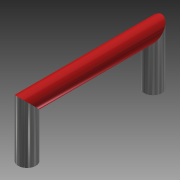
# Autodesk Inventor part: Wire 3
Saved by Autodesk Inventor 2015 (Build 190159000, 159)
## iProperties
Created: 2016-01-20
Part Number: Wire 3
Material: Generic
Document SubType Name: Modeling
Designer: Kyle
Density: 1 g/cm^3
Appearance: Default
Author: Kyle
Autodesk Inventor part; units mm, degrees
ref_plane "YZ Plane" through (0, 0, 0) normal (1, 0, 0) x (0, 1, 0)
ref_plane "XZ Plane" through (0, 0, 0) normal (0, 1, 0) x (-1, 0, 0)
ref_plane "XY Plane" through (0, 0, 0) normal (0, 0, 1) x (1, 0, 0)
sketch "Sketch1" plane through (0, 0, 0) normal (0, 0, 1) x (1, 0, 0)
  line L0 (0, 0) -> (1.0668, 0)
  line L1 (1.0668, 0) -> (1.0668, 1.0668)
  line L2 (1.0668, 1.0668) -> (0, 1.0668)
  line L3 (0, 1.0668) -> (0, 0)
  dimension "d0" = 1.0668
  dimension "d1" = 1.0668
  constraints: 8 end point, 2 parallel, 1 horizontal, 1 perpendicular
  measures "d0" distance of L1.end L2.end
  measures "d1" distance of L0.end L1.end
extrude "Extrusion1" add sketch "Sketch1" along normal blind 8.6868
sketch "Sketch2" plane through (0, 0, 0) normal (0, -1, 0) x (1, 0, 0)
  line L0 (0, 0) -> (0, 8.6868) projected
  line L1 (1.0668, 0) -> (0, 0)
  line L2 (0, 0) -> (0, 1.0668)
  line L3 (0, 1.0668) -> (1.0668, 1.0668)
  line L4 (1.0668, 1.0668) -> (1.0668, 0)
  line L5 (1.0668, 0) -> (1.0668, 8.6868) projected
  line L6 (0, 8.6868) -> (1.0668, 8.6868)
  line L7 (1.0668, 8.6868) -> (1.0668, 7.62)
  line L8 (1.0668, 7.62) -> (0, 7.62)
  line L9 (0, 7.62) -> (0, 8.6868)
  dimension "d4" = 1.0668
  dimension "d5" = 1.0668
  constraints: 16 end point, 4 parallel, 2 horizontal, 2 perpendicular, 2 point on line
  measures "d4" distance of L3.end L1.start
  measures "d5" distance of L0.end L8.end
extrude "Extrusion2" add sketch "Sketch2" along normal blind 2.54 contours L0 L3 L4 L1 | L0 L6 L5 L8
fillet "Fillet1" radius 0.5334 12 edges at (1.0668, 1.0668, 4.3434) (0, 1.0668, 4.3434) (0, 0, 4.3434) (1.0668, 0, 4.3434) (1.0668, -1.27, 1.0668) (1.0668, -0.7366, 0) (0, -0.7366, 0) (0, -1.27, 1.0668) (0, -1.27, 7.62) (1.0668, -1.27, 7.62) (0, -0.7366, 8.6868) (1.0668, -0.7366, 8.6868)
body "Solid1"
